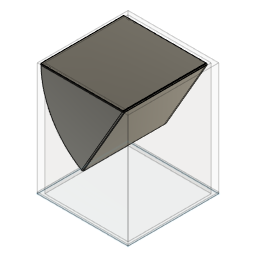
mailbox v1 (Autodesk Fusion 360 design; units mm, degrees)
Autodesk Fusion 360 part; units mm, degrees
sketch "Sketch1" plane through (0, 0, 0) normal (0, 1, 0) x (1, 0, 0)
sketch "Sketch2" plane through (0, 0, 0) normal (0, 0, 1) x (1, 0, 0)
sketch "Sketch1 (2)" plane through (0, 0, 0) normal (1, 0, 0) x (0, 1, 0) in component "Box"
sketch "Sketch2 (2)" plane through (0, 0, 0) normal (1, 0, 0) x (0, 1, 0) in component "Box"
sketch "Sketch3" plane through (0, 0, 0) normal (0, 1, 0) x (1, 0, 0) in component "Box"
sketch "Sketch4" plane through (0, 0, 0) normal (1, 0, 0) x (0, 1, 0) in component "Box"
sketch "Sketch5" plane through (0, 0, 0) normal (0, 0, 1) x (1, 0, 0) in component "Box"
  line L0 (0, 700) -> (600, 700)
  line L1 (600, 700) -> (600, 100)
  line L2 (600, 100) -> (0, 100)
  line L3 (0, 100) -> (0, 700)
  line L4 (25, 675) -> (600, 675)
  line L5 (575, 675) -> (575, 100)
  line L6 (575, 125) -> (0, 125)
  line L7 (25, 125) -> (25, 700)
  dimension "d1" = 600
  dimension "d2" = 600
  constraint horizontal L0
  constraint vertical L1
  constraint horizontal L2
  constraint vertical L3
  constraint coincident L1 L4.end
  constraint perpendicular L1 L4
  constraint coincident L4 L5.start
  constraint coincident L2 L5.end
  constraint perpendicular L2 L5
  constraint coincident L5 L6.start
  constraint coincident L3 L6.end
  constraint perpendicular L3 L6
  constraint coincident L6 L7.start
  constraint coincident L0 L7.end
  constraint perpendicular L0 L7
  measures "d1" distance of L0.start L0.end
  measures "d2" distance of L0.end L2
extrude "Extrude1" add sketch "Sketch5" along normal blind 750 contours L0 L3 L6 L7 | L0 L1 L4 L7 | L2 L3 L5 L6 | L1 L2 L4 L5 makes body 1 in component "Box"
sketch "Sketch6" plane through (0, 0, 0) normal (0, 0, 1) x (1, 0, 0) in component "Box"
  line L0 (0, 700) -> (600, 700)
  line L1 (600, 700) -> (600, 100)
  line L2 (600, 100) -> (0, 100)
  line L3 (0, 100) -> (0, 700)
  constraint horizontal L0
  constraint vertical L1
  constraint horizontal L2
  constraint vertical L3
sketch "Sketch1 (3)" plane through (0, 0, 0) normal (0, 0, 1) x (1, 0, 0) in component "Door"
  line L0 (0, 700) -> (600, 700)
  line L1 (600, 700) -> (600, 100)
  line L2 (600, 100) -> (0, 100)
  line L3 (0, 100) -> (0, 700)
  constraint horizontal L0
  constraint vertical L1
  constraint horizontal L2
  constraint vertical L3
extrude "Extrude1'" add sketch "Sketch1 (3)" along normal blind 10 separate body makes body 2 in component "Door"
sketch "Sketch1 (4)" plane through (0, 0, 10) normal (0, 0, 1) x (-1, 0, 0) in component "Upper Door (1)"
  line L0 (0, -100) -> (-600, -100)
  line L1 (-600, -100) -> (-600, -700)
  line L2 (-600, -700) -> (0, -700)
  line L3 (0, -700) -> (0, -100)
  line L4 (-25.7528, -672.0041, 1150) -> (-574.5015, -672.0041, 1150)
  line L5 (-574.5015, -672.0041, 1150) -> (-574.5015, -123.2554, 1150)
  line L6 (-574.5015, -123.2554, 1150) -> (-25.7528, -123.2554, 1150)
  line L7 (-25.7528, -123.2554, 1150) -> (-25.7528, -672.0041, 1150)
extrude "Extrude1''" add sketch "Sketch1 (4)" along normal blind 10 separate body contours L4 L5 L6 L7 in plane through (0, 0, 1160) normal (0, 0, 1) makes body 3 in component "Upper Door (1)"
sketch "Sketch2 (3)" plane through (0, 0, 0) normal (0, 1, 0) x (1, 0, 0) in component "Upper Door (1)"
  arc A0 (299.3809, -688.5589) -> (25.952, -1164.9945) centre (575.2718, -1163.5731) ccw
  line L0 (575.2718, -1163.5731) -> (299.3809, -688.5589) construction
  line L1 (575.2718, -1163.5731) -> (25.952, -1164.9945) construction
  line L2 (25.952, -1164.9945) -> (575.2718, -1163.5731)
  line L3 (299.3809, -688.5589) -> (575.2718, -1163.5731)
  dimension "d17" = 60
  constraint coincident A0.centre L0.start
  measures "d17" angle of L0 L1
extrude "Extrude2" add sketch "Sketch2 (3)" along normal blind 10 separate body makes body 4 in component "Upper Door (1)"
move_body "Move1" bodies 4 to x (1, 0, 0) y (0, 1, 0) z (0, 0, 1) at (0, 100, 0) in component "Upper Door (1)"
sketch "Sketch1 (5)" plane through (0, 0, 0) normal (1, 0, 0) x (0, 1, 0) in component "Component"
move_body "Move2" bodies 4 to x (1, 0, 0) y (0, 1, 0) z (0, 0, 1) at (0, 25, 0) in component "Upper Door (1)"
copy_body "Body->Comp1" bodies 3 removing the originals makes body 5 in component "Component'"
copy_body "Body->Comp2" bodies 4 removing the originals makes body 6 in component "Component''"
component "Box" placed x (1, 0, 0) y (0, 1, 0) z (0, 0, 1) at (0, 0, 0)
component "Door" placed x (1, 0, 0) y (0, 1, 0) z (0, 0, 1) at (0, 0, 0)
component "Upper Door (1)" placed x (1, 0, 0) y (0, 1, 0) z (0, 0, 1) at (0, 0, 0)
component "Component'" placed x (1, 0, 0) y (0, 1, 0) z (0, 0, 1) at (0, 0, 0) in component "Upper Door (1)"
component "Component''" placed x (1, 0, 0) y (0, 1, 0) z (0, 0, 1) at (0, 0, 0) in component "Upper Door (1)"
component "Component" placed x (1, 0, 0) y (0, 1, 0) z (0, 0, 1) at (0, 0, 0) in component "Upper Door (1)"
component "Component'" placed x (0.5, 0, 0.866025) y (0, 1, 0) z (-0.866025, 0, 0.5) at (1296.9221, 0, 88.7588) in component "Upper Door (1)"
component "Component''" placed x (1, 0, 0) y (0, 1, 0) z (0, 0, 1) at (0, 540, 0) in component "Component"
